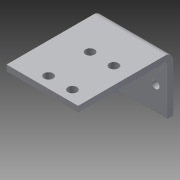
# Autodesk Inventor part: Pneumatic Piston Back Flange (Left Custom)
Saved by Autodesk Inventor 2014 (Build 180170000, 170)
## iProperties
Created: 2014-01-13
Part Number: Pneumatic Piston Back Flange (Left Custom)
Material: Aluminum 6061
Document SubType Name: Sheet Metal
Designer: Michael
Density: 2.71 g/cm^3
Sheet Metal Rule: Default
Appearance: Aluminum - Flat
Author: Michael
Autodesk Inventor part; units mm, degrees
ref_plane "YZ Plane" through (0, 0, 0) normal (1, 0, 0) x (0, 1, 0)
ref_plane "XZ Plane" through (0, 0, 0) normal (0, 1, 0) x (-1, 0, 0)
ref_plane "XY Plane" through (0, 0, 0) normal (0, 0, 1) x (1, 0, 0)
sketch "Sketch1" plane through (0, 0, 0) normal (0, 0, 1) x (1, 0, 0)
  line L0 (0, 0) -> (38.1, 0)
  line L1 (38.1, 0) -> (38.1, 25.4)
  line L2 (38.1, 25.4) -> (0, 25.4)
  line L3 (0, 25.4) -> (0, 0)
  circle A0 centre (6.35, 12.7) radius 2.0701
  circle A1 centre (31.75, 12.7) radius 2.0701
  dimension "d0" = 38.1
  dimension "d1" = 25.4
  dimension "d2" = 4.1402
  dimension "d3" = 12.7
  dimension "d4" = 6.35
  dimension "d7" = 25.4
  measures "d0" distance of L2.end L1.end
  measures "d1" distance of L1.end L0.end
  measures "d2" diameter of A0
  measures "d3" distance from line of L0 A0.centre
  measures "d4" distance from line of L3 A0.centre
  measures "d7" distance of A0.centre A1.centre
extrude "Plate1" add sketch "Sketch1" along normal blind 3.175
sketch "Sketch2" plane through (0, 26.67, 4.445) normal (0, 1, 0) x (-1, 0, 0)
  line L0 (-38.1, 0) -> (0, 0)
  line L1 (0, 0) -> (0, 46.355)
  line L2 (0, 46.355) -> (-38.1, 46.355)
  line L3 (-38.1, 46.355) -> (-38.1, 0)
  constraints: 6 end point, 1 horizontal, 1 perpendicular, 1 vertical
edge flange "Flange1" height 50.8 angle 90 thickness 3.175 bend radius 1.27 thickness toward (0, 1, 0) relief tear relief width 3.175 relief depth 1.5875 edges at (19.05, 25.4, 3.175) wall of the first edge with corners at (38.1, 26.67, 4.445) (0, 26.67, 4.445) (0, 26.67, 50.8) (38.1, 26.67, 50.8)
bend "Bend1"
corner "Corner1"
sketch "Sketch3" plane through (0, 29.845, 50.8) normal (0, 1, 0) x (1, 0, 0)
  line L0 (38.1, 46.355) -> (0, 46.355) projected
  line L1 (32.3088, 33.655) -> (13.2588, 33.655) construction
  line L2 (13.2588, 33.655) -> (13.2588, 0.381) construction
  line L3 (13.2588, 0.381) -> (32.3088, 0.381) construction
  line L4 (32.3088, 0.381) -> (32.3088, 33.655) construction
  line L5 (32.3088, 5.969) -> (13.2588, 5.969) construction
  circle A0 centre (29.1338, 5.969) radius 2.413
  line L6 (22.7838, 0.381) -> (22.7838, 33.655) construction
  circle A1 centre (16.4338, 5.969) radius 2.413
  line L7 (32.3088, 17.018) -> (13.2588, 17.018) construction
  circle A2 centre (29.1338, 28.067) radius 2.413
  circle A3 centre (16.4338, 28.067) radius 2.413
  line L8 (0, 0) -> (0, 46.355) projected
  point P0 (0, 50.8)
  dimension "d23" = 19.05
  dimension "d24" = 33.274
  dimension "d25" = 5.588
  dimension "d26" = 3.175
  dimension "d27" = 4.826
  dimension "d29" = 12.7
  dimension "d32" = 13.2588
  constraints: 14 end point, 4 centre point, 4 midpoint, 3 point on line, 3 symmetric about line, 2 parallel, 2 perpendicular, 1 horizontal, 3 other
  measures "d23" distance of L3.end L2.end
  measures "d24" distance of L2.end L1.end
  measures "d25" distance between parallel lines of L3 L5
  measures "d26" distance from line of L4 A0.centre
  measures "d27" diameter of A0
  measures "d29" distance between parallel lines of L0 L1
  measures "d32" distance between parallel lines of L8 L2
extrude "Cut1" cut sketch "Sketch3" against normal blind 3.175
equation "\"d30\" = Thickness"
equation "\"d13\" = BendReliefWidth"
equation "\"d14\" = BendReliefDepth"
equation "\"d15\" = MinimumRemnant"
equation "\"d16\" = BendRadius"
equation "\"d20\" = CornerReliefSize"
equation "\"d21\" = GapSize"
equation "\"d22\" = JacobiRadiusSize"
equation "\"BendRadius\" = Thickness"
equation "\"BendReliefWidth\" = Thickness"
equation "\"BendReliefDepth\" = 0.5 * Thickness"
equation "\"CornerReliefSize\" = 4 * Thickness"
equation "\"MinimumRemnant\" = 2 * Thickness"
equation "\"TransitionRadius\" = BendRadius"
equation "\"JacobiRadiusSize\" = BendRadius"
equation "\"GapSize\" = Thickness"
equation "\"d12\" = BendRadius"
equation "\"Thickness\" = 3.175"
body "Solid1"
